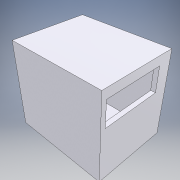
# Autodesk Inventor part: Basement
Saved by Autodesk Inventor 2018 (Build 220112000, 112)
## iProperties
Created: 2025-02-21
Part Number: Basement
Material: Všeobecné
Document SubType Name: Modeling
Designer: Jozko Mrkvicka
Density: 1 g/cm^3
Appearance: Výchozí
Author: Jozko Mrkvicka
Autodesk Inventor part; units mm, degrees
ref_plane "YZ Plane" through (0, 0, 0) normal (1, 0, 0) x (0, 1, 0)
ref_plane "XZ Plane" through (0, 0, 0) normal (0, 1, 0) x (-1, 0, 0)
ref_plane "XY Plane" through (0, 0, 0) normal (0, 0, 1) x (1, 0, 0)
sketch "Náčrt1" plane through (0, 0, 0) normal (0, 1, 0) x (-1, 0, 0)
  line L0 (-1575, 1400) -> (1575, 1400)
  line L1 (1575, 1400) -> (1575, -1400)
  line L2 (1575, -1400) -> (-1575, -1400)
  line L3 (-1575, -1400) -> (-1575, 1400)
  line L4 (-1575, 1400) -> (1575, -1400) construction
  line L5 (1575, 1400) -> (-1575, -1400) construction
  point P0 (0, 0)
  dimension "d0" = 3150
  dimension "d1" = 2800
  constraints: 12 end point, 2 midpoint, 2 parallel, 1 horizontal, 1 perpendicular
  measures "d0" distance of L1.end L2.end
  measures "d1" distance of L0.end L1.end
extrude "Vysunutí1" add sketch "Náčrt1" along normal blind 150
sketch "Náčrt2" plane through (0, 150, 0) normal (0, 1, 0) x (1, 0, 0)
  line L0 (-1575, -1400) -> (1575, -1400) projected
  line L1 (1575, -1400) -> (1575, 1400) projected
  line L2 (1575, 1400) -> (-1575, 1400) projected
  line L3 (-1575, 1400) -> (-1575, -1400) projected
  line L4 (1425, -1250) -> (-1425, -1250)
  line L5 (-1425, -1250) -> (-1425, 1250)
  line L6 (-1425, 1250) -> (1425, 1250)
  line L7 (1425, -1250) -> (-1425, 1250) construction
  line L8 (-1425, -1250) -> (1425, 1250) construction
  line L9 (1425, -1100) -> (1575, -1100)
  line L10 (1575, -1400) -> (1575, 1400) projected
  line L11 (1425, -300) -> (1575, -300)
  line L12 (1425, 1250) -> (1425, -300)
  line L13 (1425, -1100) -> (1425, -1250)
  line L14 (1575, -300) -> (1575, 1400)
  line L15 (-1575, 1400) -> (-1575, -1400) projected
  line L16 (-1575, 1400) -> (-1575, -1400)
  line L17 (-1575, -1400) -> (1575, -1400) projected
  line L18 (-1575, -1400) -> (1575, -1400)
  line L19 (1575, -1400) -> (1575, -1100)
  point P0 (0, 0)
  dimension "d4" = 2850
  dimension "d5" = 2500
  dimension "d6" = 150
  dimension "d7" = 800
  constraints: 26 end point, 5 perpendicular, 3 parallel, 2 midpoint, 2 point on line, 1 collinear, 1 horizontal, 1 vertical
  measures "d4" distance of L5.end L6.end
  measures "d5" distance of L4.end L5.end
  measures "d6" distance between parallel lines of L4 L9
  measures "d7" distance between parallel lines of L11 L9
extrude "Vysunutí2" add sketch "Náčrt2" along normal blind 2200 contours L3 L2 L1 L11 L12 L6 L5 L4 L13 L9 L0
sketch "Náčrt3" plane through (0, 2350, 0) normal (0, 1, 0) x (1, 0, 0)
  line L0 (-1575, -1400) -> (1575, -1400) projected
  line L1 (1575, -1400) -> (1575, -1100) projected
  line L2 (1575, -1100) -> (1425, -1100) projected
  line L3 (1425, -1100) -> (1425, -1250) projected
  line L4 (1425, -1250) -> (-1425, -1250) projected
  line L5 (-1425, -1250) -> (-1425, 1250) projected
  line L6 (-1425, 1250) -> (1425, 1250) projected
  line L7 (1425, 1250) -> (1425, -300) projected
  line L8 (1425, -300) -> (1575, -300) projected
  line L9 (1575, -300) -> (1575, 1400) projected
  line L10 (1575, 1400) -> (-1575, 1400) projected
  line L11 (-1575, 1400) -> (-1575, -1400) projected
  line L12 (-1575, -1400) -> (1575, -1400)
  line L13 (1575, -1400) -> (1575, 1400)
  line L14 (1575, 1400) -> (-1575, 1400)
  line L15 (-1575, 1400) -> (-1575, -1400)
  constraints: 8 end point, 2 parallel, 1 horizontal, 1 perpendicular
extrude "Vysunutí3" add sketch "Náčrt3" along normal blind 150
sketch "Náčrt4" plane through (0, 2350, 0) normal (0, -1, 0) x (1, 0, 0)
  line L0 (1575, 1100) -> (1425, 1100) projected
  line L1 (1425, 300) -> (1575, 300) projected
  line L2 (1425, 1100) -> (1575, 1100)
  line L3 (1575, 1100) -> (1575, 300)
  line L4 (1575, 300) -> (1425, 300)
  line L5 (1425, 300) -> (1425, 1100)
  point P0 (0, 0)
  constraints: 8 end point, 2 parallel, 1 horizontal, 1 perpendicular
extrude "Vysunutí4" add sketch "Náčrt4" along normal blind 300
sketch "Náčrt5" plane through (-1425, 150, 1250) normal (1, 0, 0) x (0, 0, -1)
  line L0 (2500, 0) -> (0, 0) projected
  line L1 (2500, 0) -> (2500, 2200) projected
  line L2 (0, 2200) -> (2500, 2200) projected
  line L3 (0, 0) -> (0, 2200) projected
  line L4 (1950, 1900) -> (2350, 1900)
  line L5 (2350, 1900) -> (2350, 1500)
  line L6 (2350, 1500) -> (1950, 1500)
  line L7 (1950, 1500) -> (1950, 1900)
  point P0 (1250, -150)
  dimension "d14" = 400
  dimension "d15" = 400
  dimension "d16" = 150
  dimension "d17" = 300
  constraints: 8 end point, 2 parallel, 1 horizontal, 1 perpendicular
  measures "d14" distance of L5.end L6.end
  measures "d15" distance of L4.end L5.end
  measures "d16" distance between parallel lines of L1 L5
  measures "d17" distance between parallel lines of L2 L4
extrude "Vysunutí5" cut sketch "Náčrt5" against normal up to next contours L4 L5 L6 L7
